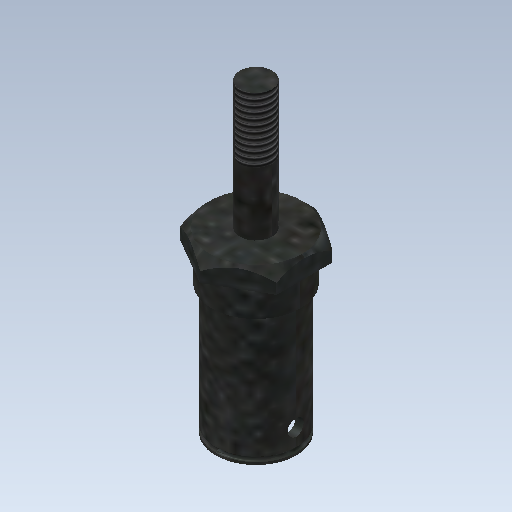
# Autodesk Inventor part: 500-126
Saved by Autodesk Inventor 2020 (Build 240168000, 168)
## iProperties
Created: 2015-04-18
Part Number: 500-126
Material: Steel
Document SubType Name: Modeling
Designer: Station9
Density: 7.85 g/cm^3
Appearance: Plate
Mass: 12.3413 g
Surface Area: 14.1806 cm^2
Volume: 1.57214 cm^3
Author: Station9
Autodesk Inventor part; units mm, degrees
ref_plane "YZ Plane" through (0, 0, 0) normal (1, 0, 0) x (0, 1, 0)
ref_plane "XZ Plane" through (0, 0, 0) normal (0, 1, 0) x (-1, 0, 0)
ref_plane "XY Plane" through (0, 0, 0) normal (0, 0, 1) x (1, 0, 0)
sketch "Sketch1" plane through (0, 0, 0) normal (0, 1, 0) x (-1, 0, 0)
  line L0 (0, -6.9282) -> (-6, -3.4641)
  line L1 (-6, -3.4641) -> (-6, 3.4641)
  line L2 (-6, 3.4641) -> (0, 6.9282)
  line L3 (0, 6.9282) -> (6, 3.4641)
  line L4 (6, 3.4641) -> (6, -3.4641)
  line L5 (6, -3.4641) -> (0, -6.9282)
  point P0 (0, 0)
  point P1 (0, 0)
  dimension "d0" = 12
  constraints: 12 end point, 1 coincident, 1 vertical, 13 other
  measures "d0" distance between parallel lines of L4 L1
extrude "Extrusion1" add sketch "Sketch1" along normal blind 2.5
sketch "Sketch2" plane through (0, 2.5, 0) normal (0, 1, 0) x (1, 0, 0)
  circle A0 centre (0, 0) radius 2
  dimension "d3" = 4
  constraints: 1 centre point, 1 coincident
  measures "d3" diameter of A0
extrude "Extrusion2" add sketch "Sketch2" along normal blind 15.8
thread "Thread1" size "M4x0.7" class "6g" standard "ANSI Metric M Profile" length 8
sketch "Sketch3" plane through (0, 0, 0) normal (0, -1, 0) x (1, 0, 0)
  circle A0 centre (0, 0) radius 5.5
  dimension "d8" = 11
  constraints: 1 centre point, 1 coincident
  measures "d8" diameter of A0
extrude "Extrusion3" add sketch "Sketch3" along normal blind 3.44
sketch "Sketch4" plane through (0, -3.44, 0) normal (0, -1, 0) x (1, 0, 0)
  circle A0 centre (0, 0) radius 5.5 projected
  circle A1 centre (0, 0) radius 5
  dimension "d11" = 10
  constraints: 1 centre point, 1 coincident
  measures "d11" diameter of A1
extrude "Extrusion4" add sketch "Sketch4" along normal blind 16 contours A1
sketch "Sketch5" plane through (0, -19.44, 0) normal (0, -1, 0) x (1, 0, 0)
  circle A0 centre (0, 0) radius 5 projected
  circle A1 centre (0, 0) radius 4
  dimension "d14" = 8
  constraints: 1 centre point, 1 coincident
  measures "d14" diameter of A1
extrude "Extrusion5" cut sketch "Sketch5" against normal blind 10 contours A1
sketch "Sketch6" plane through (0, 0, 0) normal (1, 0, 0) x (0, 1, 0)
  circle A0 centre (-16.44, 0) radius 1
  line L0 (-19.44, -4) -> (-19.44, 4) projected
  point P0 (0, 0)
  dimension "d17" = 2
  dimension "d18" = 3
  constraints: 1 centre point
  measures "d17" diameter of A0
  measures "d18" distance from line of L0 A0.centre
extrude "Extrusion6" cut sketch "Sketch6" along normal mid plane 14
sketch "Sketch7" plane through (0, 0, 0) normal (1, 0, 0) x (0, 1, 0)
  line L0 (2.5, -6.9282) -> (0, -6.9282) construction
  line L1 (0, -6.9282) -> (0, -5.5) construction
  line L2 (0, -5.5) -> (-3.44, -5.5) construction
  line L3 (-3.44, -5.5) -> (-3.44, -5) construction
  line L4 (-3.44, -5) -> (-19.44, -5) construction
  line L5 (-19.44, -5) -> (-19.44, -4) construction
  line L6 (-19.44, -4) -> (-9.44, -4) construction
  line L7 (-9.44, -4) -> (-9.44, 4) construction
  line L8 (-9.44, 4) -> (-19.44, 4) construction
  line L9 (-19.44, 4) -> (-19.44, 5) construction
  line L10 (-19.44, 5) -> (-3.44, 5) construction
  line L11 (-3.44, 5) -> (-3.44, 5.5) construction
  line L12 (-3.44, 5.5) -> (0, 5.5) construction
  line L13 (0, 5.5) -> (0, 6.9282) construction
  line L14 (0, 6.9282) -> (2.5, 6.9282) construction
  line L15 (2.5, 6.9282) -> (2.5, 2) construction
  line L16 (2.5, 2) -> (18.3, 2) construction
  line L17 (18.3, 2) -> (18.3, -2) construction
  line L18 (18.3, -2) -> (2.5, -2) construction
  line L19 (2.5, -2) -> (2.5, -6.9282) construction
  circle A0 centre (-18.84, 5) radius 0.3
  line L20 (-19.44, -4) -> (-19.44, 4) projected
  line L21 (-26.988, 0) -> (25.848, 0) projected
  point P0 (0, 0)
  dimension "d21" = 0.6
  dimension "d22" = 0.6
  constraints: 1 centre point, 1 point on line
  measures "d21" diameter of A0
  measures "d22" distance from line of L20 A0.centre
revolve "Revolution1" cut sketch "Sketch7" angle 360 about axis through (0, -10, 0) along (0, 1, 0)
sketch "Sketch8" plane through (0, 0, 0) normal (0, 0, 1) x (1, 0, 0)
  line L0 (-5.078, 3.1229) -> (-8.0424, 0.1585)
  line L1 (-8.0424, 0.1585) -> (-8.4208, 3.1229)
  line L2 (-8.4208, 3.1229) -> (-5.078, 3.1229)
  line L3 (-6, 2.5) -> (0, 2.5) projected
  line L4 (0, -26.988) -> (0, 25.848) projected
  point P0 (0, 0)
  dimension "d24" = 45
  constraints: 6 end point
  measures "d24" angle of L3 L0
revolve "Revolution2" cut sketch "Sketch8" angle 360 about axis through (0, -10, 0) along (0, 1, 0)
body "Solid1"
